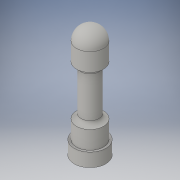
# Autodesk Inventor part: Nathan_Practice_8
Saved by Autodesk Inventor 2016 (Build 200138000, 138)
## iProperties
Created: 2017-03-09
Part Number: Nathan_Practice_8
Material: Generic
Document SubType Name: Modeling
Designer: Student
Density: 1 g/cm^3
Appearance: Default
Author: Student
Autodesk Inventor part; units mm, degrees
ref_plane "YZ Plane" through (0, 0, 0) normal (1, 0, 0) x (0, 1, 0)
ref_plane "XZ Plane" through (0, 0, 0) normal (0, 1, 0) x (-1, 0, 0)
ref_plane "XY Plane" through (0, 0, 0) normal (0, 0, 1) x (1, 0, 0)
sketch "Sketch1" plane through (0, 0, 0) normal (0, 0, 1) x (1, 0, 0)
  line L0 (-1.5, 0) -> (-3.5, 0)
  line L1 (-3.5, 0) -> (-3.5, 3)
  line L2 (-3.5, 3) -> (-3, 3)
  line L3 (-3, 3) -> (-3, 7)
  line L4 (-3, 7) -> (-2, 7)
  line L5 (-2, 7) -> (-2, 18)
  line L6 (-2, 18) -> (-3, 18)
  line L7 (-3, 18) -> (-3, 22)
  arc A0 (0, 25) -> (-3, 22) centre (0, 22) ccw
  line L8 (0, -1.5) -> (0, -2.0563)
  line L9 (0, 26.1793) -> (0, -3.524)
  arc A1 (0, 1.5) -> (-1.5, 0) centre (0, 0) ccw
  dimension "d0" = 3.5
  dimension "d1" = 3
  dimension "d2" = 0.5
  dimension "d3" = 4
  dimension "d4" = 1
  dimension "d5" = 11
  dimension "d6" = 1
  dimension "d7" = 4
  dimension "d8" = 6
  dimension "d9" = 3
  dimension "d12" = 4
  constraints: 20 end point, 5 point on circle, 5 point on line, 5 vertical, 4 horizontal, 2 centre point, 1 coincident, 1 perpendicular
  measures "d0" distance of point (0, 0) L0.end
  measures "d1" distance of L0.end L1.end
  measures "d2" distance of L1.end L2.end
  measures "d3" distance of L2.end L3.end
  measures "d4" distance of L3.end L4.end
  measures "d5" distance of L4.end L5.end
  measures "d6" distance of L5.end L6.end
  measures "d7" distance of L7.end L6.end
  measures "d8" diameter of A0
  measures "d9" diameter of A1
  measures "d12" diameter of L5 L9
revolve "Revolution1" add sketch "Sketch1" angle 360 about axis through (0, -1.5, 0) along (0, -1, 0)
fillet "Fillet1" radius 1 2 edges at (2, 7, 0) (2, 18, 0)
body "Solid1"
